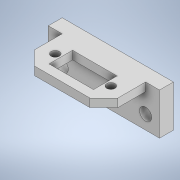
# Autodesk Inventor part: xt60_plug_mount_v2
Saved by Autodesk Inventor 2022 (Build 260153000, 153)
## iProperties
Created: 2021-10-28
Part Number: xt60_plug_mount_v2
Material: Generic
Document SubType Name: Modeling
Designer: james
Density: 1 g/cm^3
Appearance: Default
Author: james
Autodesk Inventor part; units mm, degrees
ref_plane "YZ Plane" through (0, 0, 0) normal (1, 0, 0) x (0, 1, 0)
ref_plane "XZ Plane" through (0, 0, 0) normal (0, 1, 0) x (-1, 0, 0)
ref_plane "XY Plane" through (0, 0, 0) normal (0, 0, 1) x (1, 0, 0)
sketch "Sketch1" plane through (0, 0, 0) normal (0, 0, 1) x (1, 0, 0)
  line L0 (0, 0) -> (40, 0)
  line L1 (40, 0) -> (40, 15)
  line L2 (40, 15) -> (0, 15)
  line L3 (0, 15) -> (0, 0)
  dimension "d0" = 40
  dimension "d1" = 15
  constraints: 8 end point, 2 parallel, 1 horizontal, 1 perpendicular
  measures "d0" distance of L0.start L0.end
  measures "d1" distance of L2.end L0.start
extrude "Extrusion1" add sketch "Sketch1" along normal blind 5
sketch "Sketch2" plane through (0, 15, 0) normal (0, 1, 0) x (1, 0, 0)
  line L0 (35, -5) -> (5, -5)
  line L1 (5, -5) -> (5, -20)
  line L2 (5, -20) -> (35, -20)
  line L3 (28, -16.75) -> (12, -16.75)
  line L4 (12, -16.75) -> (12, -8.25)
  line L5 (12, -8.25) -> (28, -8.25)
  circle A0 centre (30, -12.5) radius 1.5
  circle A1 centre (10, -12.5) radius 1.5
  line L6 (28, -16.75) -> (28, -8.25)
  line L7 (0, 0) -> (0, -5) projected
  line L8 (40, -5) -> (0, -5) projected
  line L9 (35, -5) -> (35, -20)
  dimension "d4" = 8.5
  dimension "d7" = 4.25
  dimension "d8" = 4.25
  dimension "d9" = 3
  dimension "d10" = 3
  dimension "d11" = 20
  dimension "d13" = 16
  dimension "d14" = 2
  dimension "d28" = 5
  dimension "d29" = 5
  dimension "d30" = 5
  dimension "d31" = 15
  dimension "d32" = 3.25
  constraints: 16 end point, 3 perpendicular, 2 centre point, 2 horizontal, 2 parallel, 1 point on line, 1 vertical
  measures "d4" distance between parallel lines of L3 L5
  measures "d7" distance from line of L3 A0.centre
  measures "d8" distance from line of L3 A1.centre
  measures "d9" diameter of A1
  measures "d10" diameter of A0
  measures "d11" distance of A1.centre A0.centre
  measures "d13" distance between parallel lines of L4 L6
  measures "d14" distance from line of A1.centre L4
  measures "d28" distance between parallel lines of L7 L1
  measures "d29" distance from line of L1 A1.centre
  measures "d30" distance from line of A0.centre L9
  measures "d31" distance of L0.start L2.end
  measures "d32" distance between parallel lines of L2 L3
extrude "Extrusion2" add sketch "Sketch2" against normal blind 3
sketch "Sketch3" plane through (0, 0, 5) normal (0, 0, 1) x (1, 0, 0)
  circle A0 centre (35, 5) radius 2.2
  circle A1 centre (5, 5) radius 2.2
  line L0 (40, 0) -> (40, 15) projected
  line L1 (0, 15) -> (0, 0) projected
  line L2 (0, 0) -> (40, 0) projected
  point P0 (40, 17)
  point P1 (0, 17)
  dimension "d17" = 4.4
  dimension "d18" = 5
  dimension "d19" = 5
  dimension "d20" = 4.4
  dimension "d21" = 5
  dimension "d22" = 5
  constraints: 2 centre point
  measures "d17" diameter of A0
  measures "d18" distance from line of A0.centre L0
  measures "d19" distance from line of L1 A1.centre
  measures "d20" diameter of A1
  measures "d21" distance from line of L2 A0.centre
  measures "d22" distance from line of L2 A1.centre
extrude "Extrusion3" cut sketch "Sketch3" against normal blind 10
chamfer "Chamfer1" distance 5 angle 45 2 edges at (5, 13.5, 20) (35, 13.5, 20)
body "Solid1"
